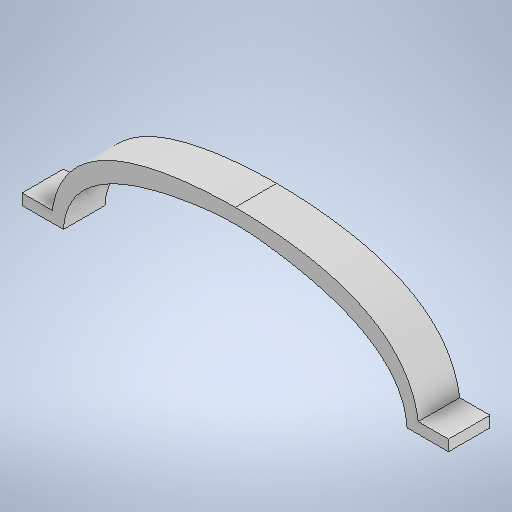
# Autodesk Inventor part: leaf spring
Saved by Autodesk Inventor 2025 (Build 290162000, 162)
## iProperties
Created: 2024-08-04
Part Number: leaf spring
Material: 일반
Document SubType Name: Modeling
Designer: unney
Density: 1 g/cm^3
Appearance: 기본값
Author: unney
Autodesk Inventor part; units mm, degrees
ref_plane "YZ Plane" through (0, 0, 0) normal (1, 0, 0) x (0, 1, 0)
ref_plane "XZ Plane" through (0, 0, 0) normal (0, 1, 0) x (-1, 0, 0)
ref_plane "XY Plane" through (0, 0, 0) normal (0, 0, 1) x (1, 0, 0)
sketch "스케치1" plane through (0, 0, 0) normal (0, 0, 1) x (1, 0, 0)
  line L0 (-30.5325, 8.0232) -> (-30.5325, 13.4232)
  line L1 (-30.5325, 13.4232) -> (-15.5325, 13.4232)
  line L2 (-30.5325, 8.0232) -> (-10.0325, 8.0232)
  line L3 (74.9675, 60.0232) -> (238.2045, 60.0232)
  line L4 (-10.1821, 0) -> (40.0685, 0)
  line L5 (74.9675, 101.3031) -> (74.9675, -114.83)
  spline S0 degree 2 poles (-15.5325, 13.4232) (-8.9113, 58.8827) (74.9675, 60.0232) knots 0 0 0 1 1 1
  spline S1 degree 2 poles (-10.0325, 8.0232) (-7.3142, 47.007) (74.9675, 53.3061) knots 0 0 0 1 1 1
  line L6 (180.4675, 8.0232) -> (180.4675, 13.4232)
  line L7 (180.4675, 13.4232) -> (165.4675, 13.4232)
  line L8 (180.4675, 8.0232) -> (159.9675, 8.0232)
  spline S2 degree 2 poles (165.4675, 13.4232) (158.8462, 58.8827) (74.9675, 60.0232) knots 0 0 0 1 1 1
  spline S3 degree 2 poles (159.9675, 8.0232) (157.2492, 47.007) (74.9675, 53.3061) knots 0 0 0 1 1 1
  point P0 (0, 0)
  point P1 (-30.5325, 10.7232)
  point P2 (2.5648, 43.0209)
  point P3 (3.7483, 33.1123)
  point P4 (147.3701, 43.0209)
  point P5 (146.1867, 33.1123)
  dimension "d1" = 20.5
  dimension "d3" = 52
  dimension "d6" = 5.4
  dimension "d8" = 15
  dimension "d11" = 105.5
  constraints: 18 end point, 6 symmetric about line, 4 horizontal, 3 vertical, 2 point on line, 1 midpoint, 1 perpendicular, 12 other
  measures "d1" distance of L0.start L2.end
  measures "d3" distance between parallel lines of L3 L2
  measures "d6" distance of L0.start L0.end
  measures "d8" distance of L0.end L1.end
  measures "d11" distance between parallel lines of L5 L0
extrude "돌출1" add sketch "스케치1" along normal blind 20.5
fillet "모깎기1" radius 120 1 edges at (74.9675, 53.3061, 10.25)
